Autodesk Fusion 360 part; units mm, degrees
(part 3 of 8)
  line L38 (161.2459, -8.965) -> (161.2459, 4.1583)
  spline S145 degree 3 poles (161.2459, 4.1583) (161.2459, 5.296) (159.7907, 5.2166) (159.7907, 5.6135) knots 0 0 0 0 1 1 1 1
  spline S146 degree 3 poles (159.7907, 5.6135) (159.7907, 5.9575) (160.0818, 6.5131) (160.2934, 6.5131) knots 0 0 0 0 1 1 1 1
  spline S147 degree 3 poles (160.2934, 6.5131) (161.3253, 6.4602) (162.6218, 6.4337) (163.9182, 6.4337) knots 0 0 0 0 1 1 1 1
  spline S148 degree 3 poles (163.9182, 6.4337) (165.2147, 6.4337) (166.4873, 6.4602) (167.5457, 6.5131) knots 0 0 0 0 1 1 1 1
  spline S149 degree 3 poles (167.5457, 6.5131) (167.7547, 6.5131) (168.0193, 5.9575) (168.0193, 5.64) knots 0 0 0 0 1 1 1 1
  spline S150 degree 3 poles (168.0193, 5.64) (168.0193, 5.2166) (166.5905, 5.296) (166.5905, 4.1583) knots 0 0 0 0 1 1 1 1
  line L39 (166.5905, 4.1583) -> (166.5905, -8.965)
  spline S151 degree 3 poles (166.5905, -8.965) (166.5905, -10.0763) (168.0193, -10.0234) (168.0193, -10.4203) knots 0 0 0 0 1 1 1 1
  spline S152 degree 3 poles (168.0193, -10.4203) (168.0193, -10.7378) (167.7547, -11.3225) (167.5457, -11.2934) knots 0 0 0 0 1 1 1 1
  spline S153 degree 3 poles (167.5457, -11.2934) (166.4873, -11.2405) (165.2147, -11.214) (163.9182, -11.214) knots 0 0 0 0 1 1 1 1
  spline S154 degree 3 poles (163.9182, -11.214) (162.6218, -11.214) (161.3253, -11.2405) (160.2934, -11.2934) knots 0 0 0 0 1 1 1 1
  spline S155 degree 3 poles (160.2934, -11.2934) (160.0818, -11.3225) (159.7907, -10.7378) (159.7907, -10.4203) knots 0 0 0 0 1 1 1 1
  spline S156 degree 3 poles (-72.8517, 6.434) (-72.0838, 6.434) (-71.3407, 6.4603) (-70.4164, 6.5133) knots 0 0 0 0 1 1 1 1
  spline S157 degree 3 poles (-70.4164, 6.5133) (-71.3407, 6.4603) (-72.0838, 6.434) (-72.8517, 6.434) knots -1 -1 -1 -1 0 0 0 0
  spline S158 degree 3 poles (9.5118, 5.6398) (9.5118, 5.2165) (8.0583, 5.2959) (8.0583, 4.1848) knots 0 0 0 0 1 1 1 1
  spline S159 degree 3 poles (8.0583, 4.1848) (8.0583, 5.2959) (9.5118, 5.2165) (9.5118, 5.6398) knots -1 -1 -1 -1 0 0 0 0
  spline S160 degree 3 poles (159.7907, -10.4203) (159.7907, -10.0234) (161.2459, -10.0763) (161.2459, -8.965) knots 0 0 0 0 1 1 1 1
  spline S161 degree 3 poles (161.2459, -8.965) (161.2459, -10.0763) (159.7907, -10.0234) (159.7907, -10.4203) knots -1 -1 -1 -1 0 0 0 0
  spline S162 degree 3 poles (88.5675, 6.5131) (88.9644, 6.4602) (90.5519, 6.4337) (92.1394, 6.4337) knots 0 0 0 0 1 1 1 1
  spline S163 degree 3 poles (92.1394, 6.4337) (90.5519, 6.4337) (88.9644, 6.4602) (88.5675, 6.5131) knots -1 -1 -1 -1 0 0 0 0
  line L40 (2.7113, 4.1848) -> (2.7113, -0.5248)
  line L41 (2.7113, -0.5248) -> (2.7113, 4.1848)
  spline S164 degree 3 poles (161.2459, -8.965) (161.2459, -10.0763) (159.7907, -10.0234) (159.7907, -10.4203) knots -1 -1 -1 -1 0 0 0 0
  spline S165 degree 3 poles (159.7907, -10.4203) (159.7907, -10.7378) (160.0818, -11.3225) (160.2934, -11.2934) knots -1 -1 -1 -1 0 0 0 0
  spline S166 degree 3 poles (160.2934, -11.2934) (161.3253, -11.2405) (162.6218, -11.214) (163.9182, -11.214) knots -1 -1 -1 -1 0 0 0 0
  spline S167 degree 3 poles (163.9182, -11.214) (165.2147, -11.214) (166.4873, -11.2405) (167.5457, -11.2934) knots -1 -1 -1 -1 0 0 0 0
  spline S168 degree 3 poles (167.5457, -11.2934) (167.7547, -11.3225) (168.0193, -10.7378) (168.0193, -10.4203) knots -1 -1 -1 -1 0 0 0 0
  spline S169 degree 3 poles (168.0193, -10.4203) (168.0193, -10.0234) (166.5905, -10.0763) (166.5905, -8.965) knots -1 -1 -1 -1 0 0 0 0
  line L42 (166.5905, -8.965) -> (166.5905, 4.1583)
  spline S170 degree 3 poles (166.5905, 4.1583) (166.5905, 5.296) (168.0193, 5.2166) (168.0193, 5.64) knots -1 -1 -1 -1 0 0 0 0
  spline S171 degree 3 poles (168.0193, 5.64) (168.0193, 5.9575) (167.7547, 6.5131) (167.5457, 6.5131) knots -1 -1 -1 -1 0 0 0 0
  spline S172 degree 3 poles (167.5457, 6.5131) (166.4873, 6.4602) (165.2147, 6.4337) (163.9182, 6.4337) knots -1 -1 -1 -1 0 0 0 0
  spline S173 degree 3 poles (163.9182, 6.4337) (162.6218, 6.4337) (161.3253, 6.4602) (160.2934, 6.5131) knots -1 -1 -1 -1 0 0 0 0
  spline S174 degree 3 poles (160.2934, 6.5131) (160.0818, 6.5131) (159.7907, 5.9575) (159.7907, 5.6135) knots -1 -1 -1 -1 0 0 0 0
  spline S175 degree 3 poles (159.7907, 5.6135) (159.7907, 5.2166) (161.2459, 5.296) (161.2459, 4.1583) knots -1 -1 -1 -1 0 0 0 0
  line L43 (161.2459, 4.1583) -> (161.2459, -8.965)
  spline S176 degree 3 poles (112.1948, 6.5131) (112.4065, 6.5395) (112.6975, 5.931) (112.6975, 5.6135) knots 0 0 0 0 1 1 1 1
  spline S177 degree 3 poles (112.6975, 5.6135) (112.6975, 5.931) (112.4065, 6.5395) (112.1948, 6.5131) knots -1 -1 -1 -1 0 0 0 0
  spline S178 degree 3 poles (109.7077, -8.9386) (109.5755, -10.0498) (111.2952, -9.9969) (111.2952, -10.4203) knots 0 0 0 0 1 1 1 1
  spline S179 degree 3 poles (111.2952, -10.4203) (111.2952, -9.9969) (109.5755, -10.0498) (109.7077, -8.9386) knots -1 -1 -1 -1 0 0 0 0
  spline S180 degree 3 poles (8.0583, -8.9652) (8.0583, -10.0763) (9.5118, -9.9969) (9.5118, -10.4202) knots 0 0 0 0 1 1 1 1
  spline S181 degree 3 poles (9.5118, -10.4202) (9.5118, -9.9969) (8.0583, -10.0763) (8.0583, -8.9652) knots -1 -1 -1 -1 0 0 0 0
  spline S182 degree 3 poles (166.5905, -8.965) (166.5905, -10.0763) (168.0193, -10.0234) (168.0193, -10.4203) knots 0 0 0 0 1 1 1 1
  spline S183 degree 3 poles (168.0193, -10.4203) (168.0193, -10.0234) (166.5905, -10.0763) (166.5905, -8.965) knots -1 -1 -1 -1 0 0 0 0
  line L44 (111.3746, 4.1583) -> (109.7077, -8.9386)
  spline S184 degree 3 poles (109.7077, -8.9386) (109.5755, -10.0498) (111.2952, -9.9969) (111.2952, -10.4203) knots 0 0 0 0 1 1 1 1
  spline S185 degree 3 poles (111.2952, -10.4203) (111.2952, -10.7378) (111.0042, -11.3225) (110.7925, -11.2934) knots 0 0 0 0 1 1 1 1
  spline S186 degree 3 poles (110.7925, -11.2934) (108.914, -11.1346) (106.9032, -11.2934) (106.0036, -11.2934) knots 0 0 0 0 1 1 1 1
  spline S187 degree 3 poles (106.0036, -11.2934) (105.104, -11.2934) (104.8394, -11.1346) (104.6542, -10.6584) knots 0 0 0 0 1 1 1 1
  line L45 (104.6542, -10.6584) -> (100.1563, 1.6977)
  line L46 (100.1563, 1.6977) -> (95.6584, -10.6584)
  spline S188 degree 3 poles (95.6584, -10.6584) (95.4732, -11.1346) (95.235, -11.2934) (94.309, -11.2934) knots 0 0 0 0 1 1 1 1
  spline S189 degree 3 poles (94.309, -11.2934) (93.4094, -11.2934) (91.6367, -11.1346) (89.7317, -11.2934) knots 0 0 0 0 1 1 1 1
  spline S190 degree 3 poles (89.7317, -11.2934) (89.52, -11.3225) (89.2555, -10.7378) (89.2555, -10.4203) knots 0 0 0 0 1 1 1 1
  spline S191 degree 3 poles (89.2555, -10.4203) (89.2555, -9.9969) (90.9223, -10.0234) (90.8165, -8.9121) knots 0 0 0 0 1 1 1 1
  line L47 (90.8165, -8.9121) -> (89.3877, 4.1583)
  spline S192 degree 3 poles (89.3877, 4.1583) (89.2819, 5.296) (88.0913, 5.2166) (88.0913, 5.6135) knots 0 0 0 0 1 1 1 1
  spline S193 degree 3 poles (88.0913, 5.6135) (88.0913, 5.931) (88.3559, 6.5395) (88.5675, 6.5131) knots 0 0 0 0 1 1 1 1
  spline S194 degree 3 poles (88.5675, 6.5131) (88.9644, 6.4602) (90.5519, 6.4337) (92.1394, 6.4337) knots 0 0 0 0 1 1 1 1
  spline S195 degree 3 poles (92.1394, 6.4337) (93.7005, 6.4337) (95.288, 6.4602) (95.6848, 6.5131) knots 0 0 0 0 1 1 1 1
  spline S196 degree 3 poles (95.6848, 6.5131) (95.8965, 6.5395) (96.1875, 5.931) (96.1875, 5.6135) knots 0 0 0 0 1 1 1 1
  spline S197 degree 3 poles (96.1875, 5.6135) (96.1875, 5.2166) (94.6265, 5.296) (94.7323, 4.1583) knots 0 0 0 0 1 1 1 1
  line L48 (94.7323, 4.1583) -> (95.7113, -4.7053)
  line L49 (95.7113, -4.7053) -> (99.7859, 6.5131)
  spline S198 degree 3 poles (99.7859, 6.5131) (100.6855, 6.4602) (101.3469, 6.4337) (102.0084, 6.4337) knots 0 0 0 0 1 1 1 1
  spline S199 degree 3 poles (102.0084, 6.4337) (102.6698, 6.4337) (103.3313, 6.4602) (104.2573, 6.5131) knots 0 0 0 0 1 1 1 1
  line L50 (104.2573, 6.5131) -> (108.2261, -4.7317)
  line L51 (108.2261, -4.7317) -> (109.3902, 4.1583)
  spline S200 degree 3 poles (109.3902, 4.1583) (109.549, 5.296) (107.9615, 5.2166) (107.9615, 5.6135) knots 0 0 0 0 1 1 1 1
  spline S201 degree 3 poles (107.9615, 5.6135) (107.9615, 5.931) (108.2261, 6.5395) (108.4377, 6.5131) knots 0 0 0 0 1 1 1 1
  spline S202 degree 3 poles (108.4377, 6.5131) (108.8346, 6.4602) (109.5755, 6.4337) (110.3163, 6.4337) knots 0 0 0 0 1 1 1 1
  spline S203 degree 3 poles (110.3163, 6.4337) (111.0571, 6.4337) (111.798, 6.4602) (112.1948, 6.5131) knots 0 0 0 0 1 1 1 1
  spline S204 degree 3 poles (112.1948, 6.5131) (112.4065, 6.5395) (112.6975, 5.931) (112.6975, 5.6135) knots 0 0 0 0 1 1 1 1
  spline S205 degree 3 poles (112.6975, 5.6135) (112.6975, 5.2166) (111.5334, 5.296) (111.3746, 4.1583) knots 0 0 0 0 1 1 1 1
  line L52 (109.7077, -8.9386) -> (111.3746, 4.1583)
  line L53 (111.3746, 4.1583) -> (109.7077, -8.9386)
  line L54 (2.7113, -0.5248) -> (0.9622, -0.5248)
  line L55 (0.9622, -0.5248) -> (2.7113, -0.5248)
  spline S206 degree 3 poles (107.9615, 5.6135) (107.9615, 5.931) (108.2261, 6.5395) (108.4377, 6.5131) knots 0 0 0 0 1 1 1 1
  spline S207 degree 3 poles (108.4377, 6.5131) (108.2261, 6.5395) (107.9615, 5.931) (107.9615, 5.6135) knots -1 -1 -1 -1 0 0 0 0
  spline S208 degree 3 poles (9.5118, -10.4202) (9.5118, -10.738) (9.2223, -11.3225) (9.0107, -11.2935) knots 0 0 0 0 1 1 1 1
  spline S209 degree 3 poles (9.0107, -11.2935) (9.2223, -11.3225) (9.5118, -10.738) (9.5118, -10.4202) knots -1 -1 -1 -1 0 0 0 0
  spline S210 degree 3 poles (214.7182, 6.5131) (215.7501, 6.4602) (217.0466, 6.4337) (218.3166, 6.4337) knots 0 0 0 0 1 1 1 1
  spline S211 degree 3 poles (218.3166, 6.4337) (217.0466, 6.4337) (215.7501, 6.4602) (214.7182, 6.5131) knots -1 -1 -1 -1 0 0 0 0
  spline S212 degree 3 poles (111.2952, -10.4203) (111.2952, -10.7378) (111.0042, -11.3225) (110.7925, -11.2934) knots 0 0 0 0 1 1 1 1
  spline S213 degree 3 poles (110.7925, -11.2934) (111.0042, -11.3225) (111.2952, -10.7378) (111.2952, -10.4203) knots -1 -1 -1 -1 0 0 0 0
  spline S214 degree 3 poles (168.0193, -10.4203) (168.0193, -10.7378) (167.7547, -11.3225) (167.5457, -11.2934) knots 0 0 0 0 1 1 1 1
  spline S215 degree 3 poles (167.5457, -11.2934) (167.7547, -11.3225) (168.0193, -10.7378) (168.0193, -10.4203) knots -1 -1 -1 -1 0 0 0 0
  spline S216 degree 3 poles (207.4951, -6.769) (207.4951, -6.5573) (208.0507, -6.2663) (208.3682, -6.2663) knots 0 0 0 0 1 1 1 1
  spline S217 degree 3 poles (208.3682, -6.2663) (208.0507, -6.2663) (207.4951, -6.5573) (207.4951, -6.769) knots -1 -1 -1 -1 0 0 0 0
  spline S218 degree 3 poles (108.4377, 6.5131) (108.8346, 6.4602) (109.5755, 6.4337) (110.3163, 6.4337) knots 0 0 0 0 1 1 1 1
  spline S219 degree 3 poles (110.3163, 6.4337) (109.5755, 6.4337) (108.8346, 6.4602) (108.4377, 6.5131) knots -1 -1 -1 -1 0 0 0 0
  line L56 (215.6707, -3.1442) -> (215.6707, -8.7798)
  line L57 (215.6707, -8.7798) -> (215.6707, -3.1442)
  line L58 (-61.1571, -8.9652) -> (-61.1571, -0.6308)
  spline S220 degree 3 poles (-61.1571, -0.6308) (-61.1571, 4.158) (-58.5644, 6.7775) (-53.9628, 6.7775) knots 0 0 0 0 0.999995 0.999995 0.999995 0.999995
  line L59 (-53.9628, 6.7775) -> (-53.9628, 6.7775)
  spline S221 degree 3 poles (-53.9628, 6.7775) (-49.3578, 6.7775) (-46.7651, 4.158) (-46.7651, -0.6308) knots 0.000005 0.000005 0.000005 0.000005 1 1 1 1
  line L60 (-46.7651, -0.6308) -> (-46.7651, -8.9652)
  spline S222 degree 3 poles (-46.7651, -8.9652) (-46.7651, -10.0765) (-45.3365, -9.9971) (-45.3365, -10.4202) knots 0 0 0 0 1 1 1 1
  spline S223 degree 3 poles (-45.3365, -10.4202) (-45.3365, -10.7379) (-45.601, -11.2935) (-45.8379, -11.2935) knots 0 0 0 0 1 1 1 1
  ellipse E6 centre (-50.1303, -11.6956) end of major axis (-56.9584, -11.7428) minor radius 0.4792 (-45.8379, -11.2935) -> (-49.4642, -11.2142) ccw
  ellipse E7 centre (-49.574, -11.5198) end of major axis (-54.89, -11.5263) minor radius 0.3056 (-49.4642, -11.2142) -> (-53.0631, -11.2935) ccw
  spline S224 degree 3 poles (-53.0631, -11.2935) (-53.2726, -11.2935) (-53.5645, -10.7379) (-53.5645, -10.4202) knots 0 0 0 0 1 1 1 1
  spline S225 degree 3 poles (-53.5645, -10.4202) (-53.5645, -9.9971) (-52.1084, -10.0765) (-52.1084, -8.9652) knots 0 0 0 0 1 1 1 1
  line L61 (-52.1084, -8.9652) -> (-52.1084, -0.3134)
  spline S226 degree 3 poles (-52.1084, -0.3134) (-52.1084, 2.7559) (-53.434, 4.3435) (-55.6798, 4.3435) knots 0 0 0 0 1 1 1 1
  spline S227 degree 3 poles (-55.6798, 4.3435) (-57.9291, 4.3435) (-59.2547, 2.7559) (-59.2547, -0.3134) knots 0 0 0 0 1 1 1 1
  line L62 (-59.2547, -0.3134) -> (-59.2547, -8.9652)
  spline S228 degree 3 poles (-59.2547, -8.9652) (-59.2547, -10.0765) (-57.7986, -9.9971) (-57.7986, -10.4202) knots 0 0 0 0 1 1 1 1
  spline S229 degree 3 poles (-57.7986, -10.4202) (-57.7986, -10.7379) (-58.0905, -11.3227) (-58.3, -11.2935) knots 0 0 0 0 1 1 1 1
  ellipse E8 centre (-60.2658, -11.5026) end of major axis (-63.0589, -11.5087) minor radius 0.2884 (-58.3, -11.2935) -> (-60.2059, -11.2142) ccw
  ellipse E9 centre (-60.1459, -11.5026) end of major axis (-62.939, -11.4965) minor radius 0.2884 (-60.2059, -11.2142) -> (-62.1118, -11.2935) ccw
  spline S230 degree 3 poles (-62.1118, -11.2935) (-62.3212, -11.3227) (-62.5342, -10.7379) (-62.5342, -10.4202) knots 0 0 0 0 1 1 1 1
  spline S231 degree 3 poles (-62.5342, -10.4202) (-62.5342, -9.9971) (-61.1571, -10.0765) (-61.1571, -8.9652) knots 0 0 0 0 1 1 1 1
  spline S232 degree 3 poles (-11.2033, 5.6928) (-11.0976, 5.2958) (-10.2518, 1.4065) (-10.2518, 1.195) knots 0 0 0 0 1 1 1 1
  spline S233 degree 3 poles (-10.2518, 1.195) (-10.2518, 1.4065) (-11.0976, 5.2958) (-11.2033, 5.6928) knots -1 -1 -1 -1 0 0 0 0
  spline S234 degree 3 poles (311.924, 6.4866) (312.3209, 6.4337) (313.1149, 6.4072) (313.9086, 6.4072) knots 0 0 0 0 1 1 1 1
  spline S235 degree 3 poles (313.9086, 6.4072) (313.1149, 6.4072) (312.3209, 6.4337) (311.924, 6.4866) knots -1 -1 -1 -1 0 0 0 0
  line L63 (-61.1571, -0.6308) -> (-61.1571, -8.9652)
  line L64 (-61.1571, -8.9652) -> (-61.1571, -0.6308)
  ellipse E10 centre (19.5885, -1.7408) end of major axis (19.5885, -11.5568) minor radius 8.5372 (12.3354, 3.4367) -> (19.0342, -11.5361) ccw
  ellipse E11 centre (19.5885, -1.7408) end of major axis (19.5885, -11.5568) minor radius 8.5372 (12.3354, 3.4367) -> (19.0342, -11.5361) ccw
  spline S236 degree 3 poles (-35.3861, -11.2138) (-38.111, -11.2138) (-40.8658, -11.2404) (-43.5907, -11.2933) knots 0 0 0 0 1 1 1 1
  spline S237 degree 3 poles (-43.5907, -11.2933) (-40.8658, -11.2404) (-38.111, -11.2138) (-35.3861, -11.2138) knots -1 -1 -1 -1 0 0 0 0
  spline S238 degree 3 poles (16.2828, -2.3771) (16.2828, 2.518) (17.3668, 4.9254) (19.7498, 4.9254) knots -1 -1 -1 -1 0 0 0 0
  spline S239 degree 3 poles (16.2828, -2.3771) (16.2828, 2.518) (17.3668, 4.9254) (19.7498, 4.9254) knots -1 -1 -1 -1 0 0 0 0
  spline S240 degree 3 poles (-37.7953, 4.1582) (-37.7953, 5.296) (-39.2508, 5.2166) (-39.2508, 5.6137) knots 0 0 0 0 1 1 1 1
  spline S241 degree 3 poles (-39.2508, 5.6137) (-39.2508, 5.2166) (-37.7953, 5.296) (-37.7953, 4.1582) knots -1 -1 -1 -1 0 0 0 0
  spline S242 degree 3 poles (18.0029, 6.6455) (17.2638, 6.85) (16.5713, 7.0359) (15.9755, 7.1529) knots 0 0 0 0 0.594925 0.594925 0.594925 0.594925
  spline S243 degree 3 poles (15.9755, 7.1529) (16.5713, 7.0359) (17.2638, 6.85) (18.0029, 6.6455) knots -0.594925 -0.594925 -0.594925 -0.594925 0 0 0 0
  spline S244 degree 3 poles (-43.5907, -11.2933) (-44.1191, -11.3225) (-44.4381, -11.161) (-44.4381, -10.6848) knots 0 0 0 0 1 1 1 1
  spline S245 degree 3 poles (-44.4381, -10.6848) (-44.4381, -11.161) (-44.1191, -11.3225) (-43.5907, -11.2933) knots -1 -1 -1 -1 0 0 0 0
  spline S246 degree 3 poles (24.3546, 13.0748) (26.2837, 13.0748) (27.8455, 11.3814) (27.8455, 9.3176) knots 0 0 0 0 1 1 1 1
  spline S247 degree 3 poles (27.8455, 9.3176) (27.8455, 11.3814) (26.2837, 13.0748) (24.3546, 13.0748) knots -1 -1 -1 -1 0 0 0 0
  spline S248 degree 3 poles (-39.2508, 5.6137) (-39.2508, 5.931) (-38.9584, 6.5132) (-38.7457, 6.5132) knots 0 0 0 0 1 1 1 1
  spline S249 degree 3 poles (-38.7457, 6.5132) (-38.9584, 6.5132) (-39.2508, 5.931) (-39.2508, 5.6137) knots -1 -1 -1 -1 0 0 0 0
  spline S250 degree 3 poles (15.9755, 7.1529) (15.5699, 7.2326) (15.2092, 7.2804) (14.9092, 7.2804) knots 0.594925 0.594925 0.594925 0.594925 1 1 1 1
  spline S251 degree 3 poles (14.9092, 7.2804) (15.2092, 7.2804) (15.5699, 7.2326) (15.9755, 7.1529) knots -1 -1 -1 -1 -0.594925 -0.594925 -0.594925 -0.594925
  spline S252 degree 3 poles (-44.4381, -10.6848) (-44.4381, -10.1292) (-44.0427, -6.4516) (-44.0427, -6.2399) knots 0 0 0 0 1 1 1 1
  spline S253 degree 3 poles (-44.0427, -6.2399) (-44.0427, -6.4516) (-44.4381, -10.1292) (-44.4381, -10.6848) knots -1 -1 -1 -1 0 0 0 0
  spline S254 degree 3 poles (-38.7457, 6.5132) (-37.7156, 6.46) (-36.4196, 6.4338) (-35.1236, 6.4338) knots 0 0 0 0 1 1 1 1
  spline S255 degree 3 poles (-35.1236, 6.4338) (-36.4196, 6.4338) (-37.7156, 6.46) (-38.7457, 6.5132) knots -1 -1 -1 -1 0 0 0 0
  spline S256 degree 3 poles (21.3624, 10.7728) (21.3624, 11.8842) (22.739, 13.0748) (24.3546, 13.0748) knots 0 0 0 0 1 1 1 1
  spline S257 degree 3 poles (24.3546, 13.0748) (22.739, 13.0748) (21.3624, 11.8842) (21.3624, 10.7728) knots -1 -1 -1 -1 0 0 0 0
  spline S258 degree 3 poles (-27.1849, -11.2933) (-29.9364, -11.2404) (-32.6613, -11.2138) (-35.3861, -11.2138) knots 0 0 0 0 1 1 1 1
  spline S259 degree 3 poles (-35.3861, -11.2138) (-32.6613, -11.2138) (-29.9364, -11.2404) (-27.1849, -11.2933) knots -1 -1 -1 -1 0 0 0 0
  spline S260 degree 3 poles (14.9092, 7.2804) (13.9565, 7.2804) (13.637, 6.8569) (13.637, 6.2749) knots 0 0 0 0 1 1 1 1
  spline S261 degree 3 poles (13.637, 6.2749) (13.637, 6.8569) (13.9565, 7.2804) (14.9092, 7.2804) knots -1 -1 -1 -1 0 0 0 0
  spline S262 degree 3 poles (22.8466, 8.9736) (22.2105, 8.9736) (21.3624, 9.9262) (21.3624, 10.7728) knots 0 0 0 0 1 1 1 1
  spline S263 degree 3 poles (21.3624, 10.7728) (21.3624, 9.9262) (22.2105, 8.9736) (22.8466, 8.9736) knots -1 -1 -1 -1 0 0 0 0
  spline S264 degree 3 poles (-35.1236, 6.4338) (-33.8243, 6.4338) (-32.5549, 6.46) (-31.4982, 6.5132) knots 0 0 0 0 1 1 1 1
  spline S265 degree 3 poles (-31.4982, 6.5132) (-32.5549, 6.46) (-33.8243, 6.4338) (-35.1236, 6.4338) knots -1 -1 -1 -1 0 0 0 0
  spline S266 degree 3 poles (13.637, 6.2749) (13.637, 6.2221) (13.5056, 6.1955) (13.3205, 6.1955) knots 0 0 0 0 1 1 1 1
  spline S267 degree 3 poles (13.3205, 6.1955) (13.5056, 6.1955) (13.637, 6.2221) (13.637, 6.2749) knots -1 -1 -1 -1 0 0 0 0
  spline S268 degree 3 poles (24.0351, 9.5293) (23.3482, 9.5293) (23.0556, 8.9736) (22.8466, 8.9736) knots 0 0 0 0 1 1 1 1
  spline S269 degree 3 poles (22.8466, 8.9736) (23.0556, 8.9736) (23.3482, 9.5293) (24.0351, 9.5293) knots -1 -1 -1 -1 0 0 0 0
  spline S270 degree 3 poles (-26.2578, -10.4731) (-26.3641, -11.161) (-26.63, -11.3225) (-27.1849, -11.2933) knots 0 0 0 0 1 1 1 1
  spline S271 degree 3 poles (-27.1849, -11.2933) (-26.63, -11.3225) (-26.3641, -11.161) (-26.2578, -10.4731) knots -1 -1 -1 -1 0 0 0 0
  spline S272 degree 3 poles (109.3902, 4.1583) (109.549, 5.296) (107.9615, 5.2166) (107.9615, 5.6135) knots 0 0 0 0 1 1 1 1
  spline S273 degree 3 poles (107.9615, 5.6135) (107.9615, 5.2166) (109.549, 5.296) (109.3902, 4.1583) knots -1 -1 -1 -1 0 0 0 0
  spline S274 degree 3 poles (215.6707, -8.7798) (215.6707, -9.4148) (215.3268, -9.3619) (213.7393, -9.3619) knots -1 -1 -1 -1 0 0 0 0
  spline S275 degree 3 poles (213.7393, -9.3619) (208.9503, -9.3619) (208.8709, -6.2663) (208.3682, -6.2663) knots -1 -1 -1 -1 0 0 0 0
  spline S276 degree 3 poles (208.3682, -6.2663) (208.0507, -6.2663) (207.4951, -6.5573) (207.4951, -6.769) knots -1 -1 -1 -1 0 0 0 0
  spline S277 degree 3 poles (207.4951, -6.769) (207.4951, -6.9807) (207.0718, -10.1028) (207.0718, -10.6848) knots -1 -1 -1 -1 0 0 0 0
  spline S278 degree 3 poles (207.0718, -10.6848) (207.0718, -11.1611) (207.3893, -11.3225) (207.9184, -11.2934) knots -1 -1 -1 -1 0 0 0 0
  spline S279 degree 3 poles (207.9184, -11.2934) (209.8764, -11.2405) (212.628, -11.214) (215.3532, -11.214) knots -1 -1 -1 -1 0 0 0 0
  spline S280 degree 3 poles (215.3532, -11.214) (217.7874, -11.214) (220.1951, -11.2405) (221.9414, -11.2934) knots -1 -1 -1 -1 0 0 0 0
  spline S281 degree 3 poles (221.9414, -11.2934) (222.1795, -11.2934) (222.4441, -10.7113) (222.4441, -10.3938) knots -1 -1 -1 -1 0 0 0 0
  spline S282 degree 3 poles (222.4441, -10.3938) (222.4441, -9.9969) (221.0153, -10.0763) (221.0153, -8.9386) knots -1 -1 -1 -1 0 0 0 0
  line L65 (221.0153, -8.9386) -> (221.0153, 4.1583)
  spline S283 degree 3 poles (221.0153, 4.1583) (221.0153, 5.296) (222.4441, 5.2166) (222.4441, 5.64) knots -1 -1 -1 -1 0 0 0 0
  spline S284 degree 3 poles (222.4441, 5.64) (222.4441, 5.9575) (222.1795, 6.5131) (221.9414, 6.5131) knots -1 -1 -1 -1 0 0 0 0
  spline S285 degree 3 poles (221.9414, 6.5131) (220.883, 6.4602) (219.613, 6.4337) (218.3166, 6.4337) knots -1 -1 -1 -1 0 0 0 0
  spline S286 degree 3 poles (218.3166, 6.4337) (217.0466, 6.4337) (215.7501, 6.4602) (214.7182, 6.5131) knots -1 -1 -1 -1 0 0 0 0
  spline S287 degree 3 poles (214.7182, 6.5131) (214.5066, 6.5131) (214.2155, 5.9575) (214.2155, 5.6135) knots -1 -1 -1 -1 0 0 0 0
  spline S288 degree 3 poles (214.2155, 5.6135) (214.2155, 5.2166) (215.6707, 5.296) (215.6707, 4.1583) knots -1 -1 -1 -1 0 0 0 0
  line L66 (215.6707, 4.1583) -> (215.6707, -1.2921)
  line L67 (215.6707, -1.2921) -> (213.8186, -1.2392)
  spline S289 degree 3 poles (213.8186, -1.2392) (211.6491, -1.1863) (211.8078, 1.5389) (211.0141, 1.5389) knots -1 -1 -1 -1 0 0 0 0
  spline S290 degree 3 poles (211.0141, 1.5389) (210.6966, 1.5389) (210.1145, 1.2479) (210.1145, 1.0362) knots -1 -1 -1 -1 0 0 0 0
  spline S291 degree 3 poles (210.1145, 1.0362) (210.2468, -1.1334) (210.2468, -3.303) (210.1145, -5.4725) knots -1 -1 -1 -1 0 0 0 0
  spline S292 degree 3 poles (210.1145, -5.4725) (210.1145, -5.6842) (210.6966, -5.9753) (211.0141, -5.9753) knots -1 -1 -1 -1 0 0 0 0
  spline S293 degree 3 poles (211.0141, -5.9753) (211.8078, -5.9753) (211.6491, -3.25) (213.8186, -3.1971) knots -1 -1 -1 -1 0 0 0 0
  line L68 (213.8186, -3.1971) -> (215.6707, -3.1442)
  line L69 (215.6707, -3.1442) -> (215.6707, -8.7798)
  line L70 (100.1563, 1.6977) -> (104.6542, -10.6584)
  line L71 (104.6542, -10.6584) -> (100.1563, 1.6977)
  spline S294 degree 3 poles (313.9086, 6.4072) (314.7024, 6.4072) (315.4961, 6.4337) (315.893, 6.4866) knots 0 0 0 0 1 1 1 1
  spline S295 degree 3 poles (315.893, 6.4866) (315.4961, 6.4337) (314.7024, 6.4072) (313.9086, 6.4072) knots -1 -1 -1 -1 0 0 0 0
  spline S296 degree 3 poles (-17.4217, 6.7775) (-14.9356, 6.7775) (-14.1155, 6.2749) (-13.1896, 6.2749) knots 0 0 0 0 1 1 1 1
  spline S297 degree 3 poles (-13.1896, 6.2749) (-14.1155, 6.2749) (-14.9356, 6.7775) (-17.4217, 6.7775) knots -1 -1 -1 -1 0 0 0 0
  line L72 (-61.1571, -0.6308) -> (-61.1571, -8.9652)
  spline S298 degree 3 poles (-61.1571, -8.9652) (-61.1571, -10.0765) (-62.5342, -9.9971) (-62.5342, -10.4202) knots -1 -1 -1 -1 0 0 0 0
  spline S299 degree 3 poles (-62.5342, -10.4202) (-62.5342, -10.7379) (-62.3212, -11.3227) (-62.1118, -11.2935) knots -1 -1 -1 -1 0 0 0 0
  ellipse E12 centre (-60.1459, -11.5026) end of major axis (-62.939, -11.4965) minor radius 0.2884 (-60.2059, -11.2142) -> (-62.1118, -11.2935) ccw
  ellipse E13 centre (-60.2658, -11.5026) end of major axis (-63.0589, -11.5087) minor radius 0.2884 (-58.3, -11.2935) -> (-60.2059, -11.2142) ccw
  spline S300 degree 3 poles (-58.3, -11.2935) (-58.0905, -11.3227) (-57.7986, -10.7379) (-57.7986, -10.4202) knots -1 -1 -1 -1 0 0 0 0
  spline S301 degree 3 poles (-57.7986, -10.4202) (-57.7986, -9.9971) (-59.2547, -10.0765) (-59.2547, -8.9652) knots -1 -1 -1 -1 0 0 0 0
  line L73 (-59.2547, -8.9652) -> (-59.2547, -0.3134)
  spline S302 degree 3 poles (-59.2547, -0.3134) (-59.2547, 2.7559) (-57.9291, 4.3435) (-55.6798, 4.3435) knots -1 -1 -1 -1 0 0 0 0
  spline S303 degree 3 poles (-55.6798, 4.3435) (-53.434, 4.3435) (-52.1084, 2.7559) (-52.1084, -0.3134) knots -1 -1 -1 -1 0 0 0 0
  line L74 (-52.1084, -0.3134) -> (-52.1084, -8.9652)
  spline S304 degree 3 poles (-52.1084, -8.9652) (-52.1084, -10.0765) (-53.5645, -9.9971) (-53.5645, -10.4202) knots -1 -1 -1 -1 0 0 0 0
  spline S305 degree 3 poles (-53.5645, -10.4202) (-53.5645, -10.7379) (-53.2726, -11.2935) (-53.0631, -11.2935) knots -1 -1 -1 -1 0 0 0 0
  ellipse E14 centre (-49.574, -11.5198) end of major axis (-54.89, -11.5263) minor radius 0.3056 (-49.4642, -11.2142) -> (-53.0631, -11.2935) ccw
  ellipse E15 centre (-50.1303, -11.6956) end of major axis (-56.9584, -11.7428) minor radius 0.4792 (-45.8379, -11.2935) -> (-49.4642, -11.2142) ccw
  spline S306 degree 3 poles (-45.8379, -11.2935) (-45.601, -11.2935) (-45.3365, -10.7379) (-45.3365, -10.4202) knots -1 -1 -1 -1 0 0 0 0
  spline S307 degree 3 poles (-45.3365, -10.4202) (-45.3365, -9.9971) (-46.7651, -10.0765) (-46.7651, -8.9652) knots -1 -1 -1 -1 0 0 0 0
  line L75 (-46.7651, -8.9652) -> (-46.7651, -0.6308)
  spline S308 degree 3 poles (-46.7651, -0.6308) (-46.7651, 4.158) (-49.3578, 6.7775) (-53.9628, 6.7775) knots -1 -1 -1 -1 -0.000005 -0.000005 -0.000005 -0.000005
  line L76 (-53.9628, 6.7775) -> (-53.9628, 6.7775)
  spline S309 degree 3 poles (-53.9628, 6.7775) (-58.5644, 6.7775) (-61.1571, 4.158) (-61.1571, -0.6308) knots -0.999995 -0.999995 -0.999995 -0.999995 0 0 0 0
  line L77 (299.0115, 4.1318) -> (304.277, -10.6848)
  line L78 (304.277, -10.6848) -> (299.0115, 4.1318)
  spline S310 degree 3 poles (-115.636, 5.6133) (-115.636, 5.2164) (-116.5623, 5.0843) (-117.1979, 4.132) knots 0 0 0 0 1 1 1 1
  spline S311 degree 3 poles (-117.1979, 4.132) (-116.5623, 5.0843) (-115.636, 5.2164) (-115.636, 5.6133) knots -1 -1 -1 -1 0 0 0 0
  spline S312 degree 3 poles (110.7925, -11.2934) (108.914, -11.1346) (106.9032, -11.2934) (106.0036, -11.2934) knots 0 0 0 0 1 1 1 1
  spline S313 degree 3 poles (106.0036, -11.2934) (106.9032, -11.2934) (108.914, -11.1346) (110.7925, -11.2934) knots -1 -1 -1 -1 0 0 0 0
  line L79 (-64.9913, -8.9383) -> (-70.4164, 6.5133)
  spline S314 degree 3 poles (-70.4164, 6.5133) (-71.3407, 6.4603) (-72.0838, 6.434) (-72.8517, 6.434) knots -1 -1 -1 -1 0 0 0 0
  spline S315 degree 3 poles (-72.8517, 6.434) (-73.5911, 6.434) (-74.3591, 6.4603) (-75.2585, 6.5133) knots -1 -1 -1 -1 0 0 0 0
  line L80 (-75.2585, 6.5133) -> (-80.6801, -8.9383)
  spline S316 degree 3 poles (-80.6801, -8.9383) (-81.0534, -9.9967) (-82.2692, -9.9704) (-82.2692, -10.3935) knots -1 -1 -1 -1 0 0 0 0
  spline S317 degree 3 poles (-82.2692, -10.3935) (-82.2692, -10.7109) (-81.9777, -11.2933) (-81.768, -11.2666) knots -1 -1 -1 -1 0 0 0 0
  spline S318 degree 3 poles (-81.768, -11.2666) (-81.3698, -11.2136) (-80.577, -11.1902) (-79.7806, -11.1902) knots -1 -1 -1 -1 0 0 0 0
  spline S319 degree 3 poles (-79.7806, -11.1902) (-78.9878, -11.1902) (-78.1951, -11.2136) (-77.772, -11.2666) knots -1 -1 -1 -1 0 0 0 0
  spline S320 degree 3 poles (-77.772, -11.2666) (-77.5587, -11.2933) (-77.2956, -10.7109) (-77.2956, -10.3935) knots -1 -1 -1 -1 0 0 0 0
  spline S321 degree 3 poles (-77.2956, -10.3935) (-77.2956, -9.9704) (-78.9629, -9.9967) (-78.5932, -8.9383) knots -1 -1 -1 -1 0 0 0 0
  line L81 (-78.5932, -8.9383) -> (-74.6506, 2.4388)
  line L82 (-74.6506, 2.4388) -> (-70.6626, -9.3268)
  spline S322 degree 3 poles (-70.6626, -9.3268) (-70.7276, -9.7127) (-71.1604, -9.8874) (-71.5166, -10.0352) knots -0.858522 -0.858522 -0.858522 -0.858522 -0.365068 -0.365068 -0.365068 -0.365068
  spline S323 degree 5 poles (-71.5166, -10.0352) (-71.5378, -10.0556) (-71.6088, -10.1255) (-71.7201, -10.2417) (-71.821, -10.3613) (-71.8986, -10.4733) (-71.9463, -10.562) (-71.967, -10.6087) (-71.9703, -10.6166) knots -0.740882 -0.740882 -0.740882 -0.740882 -0.740882 -0.740882 -0.7 -0.6 -0.5 -0.479543 -0.479543 -0.479543 -0.479543 -0.479543 -0.479543
  spline S324 degree 3 poles (-71.9703, -10.6166) (-71.9088, -10.861) (-71.7664, -11.1349) (-71.625, -11.231) knots -0.790921 -0.790921 -0.790921 -0.790921 -0.15171 -0.15171 -0.15171 -0.15171
  spline S325 degree 5 poles (-71.625, -11.231) (-71.6062, -11.2385) (-71.5869, -11.2458) (-71.567, -11.2529) (-71.5465, -11.2598) (-71.5256, -11.2666) knots -0.041035 -0.041035 -0.041035 -0.041035 -0.041035 -0.041035 0 0 0 0 0 0
  spline S326 degree 3 poles (-71.5256, -11.2666) (-70.4697, -11.2136) (-69.0939, -11.1902) (-67.7181, -11.1902) knots -1 -1 -1 -1 0 0 0 0
  spline S327 degree 3 poles (-67.7181, -11.1902) (-66.3422, -11.1902) (-64.9664, -11.2136) (-63.907, -11.2666) knots -1 -1 -1 -1 0 0 0 0
  spline S328 degree 5 poles (-63.907, -11.2666) (-63.8508, -11.2222) (-63.7825, -11.1656) (-63.7203, -11.1105) (-63.6642, -11.057) (-63.6143, -11.005) (-63.6031, -10.9931) knots -1 -1 -1 -1 -1 -1 -0.933333 -0.913312 -0.913312 -0.913312 -0.913312 -0.913312 -0.913312
  spline S329 degree 3 poles (-63.6031, -10.9931) (-63.4913, -10.8075) (-63.4057, -10.5655) (-63.4057, -10.3935) knots -0.541892 -0.541892 -0.541892 -0.541892 0 0 0 0
  spline S330 degree 5 poles (-63.4057, -10.3935) (-63.4069, -10.3913) (-63.4229, -10.3621) (-63.4609, -10.3077) (-63.5364, -10.2311) (-63.6683, -10.1358) (-63.8597, -10.0252) (-64.0239, -9.9353) (-64.1456, -9.8652) (-64.2235, -9.8172) (-64.2599, -9.7941) knots -0.672047 -0.672047 -0.672047 -0.672047 -0.672047 -0.672047 -0.666667 -0.6 -0.533333 -0.466667 -0.4 -0.340251 -0.340251 -0.340251 -0.340251 -0.340251 -0.340251
  spline S331 degree 3 poles (-64.2599, -9.7941) (-64.5406, -9.6256) (-64.8201, -9.3864) (-64.9744, -8.9843) knots -0.406295 -0.406295 -0.406295 -0.406295 -0.014693 -0.014693 -0.014693 -0.014693
  spline S332 degree 5 poles (-64.9744, -8.9843) (-64.9779, -8.9752) (-64.9814, -8.966) (-64.9848, -8.9569) (-64.9881, -8.9476) (-64.9913, -8.9383) knots -0.014784 -0.014784 -0.014784 -0.014784 -0.014784 -0.014784 0 0 0 0 0 0
  ellipse E16 centre (-49.574, -11.5198) end of major axis (-54.89, -11.5263) minor radius 0.3056 (-49.4642, -11.2142) -> (-53.0631, -11.2935) ccw
  ellipse E17 centre (-49.574, -11.5198) end of major axis (-54.89, -11.5263) minor radius 0.3056 (-49.4642, -11.2142) -> (-53.0631, -11.2935) ccw
  spline S333 degree 3 poles (-116.6669, -11.2934) (-117.725, -11.2403) (-119.2598, -11.2139) (-120.8217, -11.2139) knots 0 0 0 0 1 1 1 1
  spline S334 degree 3 poles (-120.8217, -11.2139) (-119.2598, -11.2139) (-117.725, -11.2403) (-116.6669, -11.2934) knots -1 -1 -1 -1 0 0 0 0
  spline S335 degree 3 poles (2.7113, 4.1848) (2.7113, 5.2959) (1.2548, 5.2165) (1.2548, 5.6398) knots 0 0 0 0 1 1 1 1
  spline S336 degree 3 poles (1.2548, 5.6398) (1.2548, 5.2165) (2.7113, 5.2959) (2.7113, 4.1848) knots -1 -1 -1 -1 0 0 0 0
  spline S337 degree 3 poles (-82.2692, -10.3935) (-82.2692, -9.9704) (-81.0534, -9.9967) (-80.6801, -8.9383) knots 0 0 0 0 1 1 1 1
  spline S338 degree 3 poles (-80.6801, -8.9383) (-81.0534, -9.9967) (-82.2692, -9.9704) (-82.2692, -10.3935) knots -1 -1 -1 -1 0 0 0 0
  spline S339 degree 3 poles (1.4134, -2.4299) (1.8367, -2.4299) (2.7113, -2.377) (2.7113, -3.0383) knots -1 -1 -1 -1 0 0 0 0
  spline S340 degree 3 poles (1.4134, -2.4299) (1.8367, -2.4299) (2.7113, -2.377) (2.7113, -3.0383) knots -1 -1 -1 -1 0 0 0 0
  spline S341 degree 3 poles (-2.6606, -5.949) (-2.6606, -3.8323) (-1.2321, -2.4299) (1.4134, -2.4299) knots -1 -1 -1 -1 0 0 0 0
  spline S342 degree 3 poles (-2.6606, -5.949) (-2.6606, -3.8323) (-1.2321, -2.4299) (1.4134, -2.4299) knots -1 -1 -1 -1 0 0 0 0
  spline S343 degree 5 poles (-64.2599, -9.7941) (-64.2235, -9.8172) (-64.1456, -9.8652) (-64.0239, -9.9353) (-63.8597, -10.0252) (-63.6683, -10.1358) (-63.5364, -10.2311) (-63.4609, -10.3077) (-63.4229, -10.3621) (-63.4069, -10.3913) (-63.4057, -10.3935) knots 0.340251 0.340251 0.340251 0.340251 0.340251 0.340251 0.4 0.466667 0.533333 0.6 0.666667 0.672047 0.672047 0.672047 0.672047 0.672047 0.672047
  spline S344 degree 5 poles (-63.4057, -10.3935) (-63.4069, -10.3913) (-63.4229, -10.3621) (-63.4609, -10.3077) (-63.5364, -10.2311) (-63.6683, -10.1358) (-63.8597, -10.0252) (-64.0239, -9.9353) (-64.1456, -9.8652) (-64.2235, -9.8172) (-64.2599, -9.7941) knots -0.672047 -0.672047 -0.672047 -0.672047 -0.672047 -0.672047 -0.666667 -0.6 -0.533333 -0.466667 -0.4 -0.340251 -0.340251 -0.340251 -0.340251 -0.340251 -0.340251
  spline S345 degree 3 poles (-46.7651, -8.9652) (-46.7651, -10.0765) (-45.3365, -9.9971) (-45.3365, -10.4202) knots 0 0 0 0 1 1 1 1
  spline S346 degree 3 poles (-45.3365, -10.4202) (-45.3365, -9.9971) (-46.7651, -10.0765) (-46.7651, -8.9652) knots -1 -1 -1 -1 0 0 0 0
  line L83 (-59.2547, -8.9652) -> (-59.2547, -0.3134)
  line L84 (-59.2547, -0.3134) -> (-59.2547, -8.9652)
  spline S347 degree 3 poles (-45.3365, -10.4202) (-45.3365, -10.7379) (-45.601, -11.2935) (-45.8379, -11.2935) knots 0 0 0 0 1 1 1 1
  spline S348 degree 3 poles (-45.8379, -11.2935) (-45.601, -11.2935) (-45.3365, -10.7379) (-45.3365, -10.4202) knots -1 -1 -1 -1 0 0 0 0
  spline S349 degree 3 poles (-71.5166, -10.0352) (-71.1604, -9.8874) (-70.7276, -9.7127) (-70.6626, -9.3268) knots 0.365068 0.365068 0.365068 0.365068 0.858522 0.858522 0.858522 0.858522
  spline S350 degree 3 poles (-70.6626, -9.3268) (-70.7276, -9.7127) (-71.1604, -9.8874) (-71.5166, -10.0352) knots -0.858522 -0.858522 -0.858522 -0.858522 -0.365068 -0.365068 -0.365068 -0.365068
  spline S351 degree 3 poles (-55.6798, 4.3435) (-57.9291, 4.3435) (-59.2547, 2.7559) (-59.2547, -0.3134) knots 0 0 0 0 1 1 1 1
  spline S352 degree 3 poles (-59.2547, -0.3134) (-59.2547, 2.7559) (-57.9291, 4.3435) (-55.6798, 4.3435) knots -1 -1 -1 -1 0 0 0 0
  spline S353 degree 3 poles (-75.2585, 6.5133) (-74.3591, 6.4603) (-73.5911, 6.434) (-72.8517, 6.434) knots 0 0 0 0 1 1 1 1
  spline S354 degree 3 poles (-72.8517, 6.434) (-73.5911, 6.434) (-74.3591, 6.4603) (-75.2585, 6.5133) knots -1 -1 -1 -1 0 0 0 0
  spline S355 degree 5 poles (-64.9913, -8.9383) (-64.9881, -8.9476) (-64.9848, -8.9569) (-64.9814, -8.966) (-64.9779, -8.9752) (-64.9744, -8.9843) knots 0 0 0 0 0 0 0.014784 0.014784 0.014784 0.014784 0.014784 0.014784
  spline S356 degree 5 poles (-64.9744, -8.9843) (-64.9779, -8.9752) (-64.9814, -8.966) (-64.9848, -8.9569) (-64.9881, -8.9476) (-64.9913, -8.9383) knots -0.014784 -0.014784 -0.014784 -0.014784 -0.014784 -0.014784 0 0 0 0 0 0
  ellipse E18 centre (-50.1303, -11.6956) end of major axis (-56.9584, -11.7428) minor radius 0.4792 (-45.8379, -11.2935) -> (-49.4642, -11.2142) ccw
  ellipse E19 centre (-50.1303, -11.6956) end of major axis (-56.9584, -11.7428) minor radius 0.4792 (-45.8379, -11.2935) -> (-49.4642, -11.2142) ccw
  line L85 (-70.4164, 6.5133) -> (-64.9913, -8.9383)
  spline S357 degree 5 poles (-64.9913, -8.9383) (-64.9881, -8.9476) (-64.9848, -8.9569) (-64.9814, -8.966) (-64.9779, -8.9752) (-64.9744, -8.9843) knots 0 0 0 0 0 0 0.014784 0.014784 0.014784 0.014784 0.014784 0.014784
  spline S358 degree 3 poles (-64.9744, -8.9843) (-64.8201, -9.3864) (-64.5406, -9.6256) (-64.2599, -9.7941) knots 0.014693 0.014693 0.014693 0.014693 0.406295 0.406295 0.406295 0.406295
  spline S359 degree 5 poles (-64.2599, -9.7941) (-64.2235, -9.8172) (-64.1456, -9.8652) (-64.0239, -9.9353) (-63.8597, -10.0252) (-63.6683, -10.1358) (-63.5364, -10.2311) (-63.4609, -10.3077) (-63.4229, -10.3621) (-63.4069, -10.3913) (-63.4057, -10.3935) knots 0.340251 0.340251 0.340251 0.340251 0.340251 0.340251 0.4 0.466667 0.533333 0.6 0.666667 0.672047 0.672047 0.672047 0.672047 0.672047 0.672047
  spline S360 degree 3 poles (-63.4057, -10.3935) (-63.4057, -10.5655) (-63.4913, -10.8075) (-63.6031, -10.9931) knots 0 0 0 0 0.541892 0.541892 0.541892 0.541892
  spline S361 degree 5 poles (-63.6031, -10.9931) (-63.6143, -11.005) (-63.6642, -11.057) (-63.7203, -11.1105) (-63.7825, -11.1656) (-63.8508, -11.2222) (-63.907, -11.2666) knots 0.913312 0.913312 0.913312 0.913312 0.913312 0.913312 0.933333 1 1 1 1 1 1
  spline S362 degree 3 poles (-63.907, -11.2666) (-64.9664, -11.2136) (-66.3422, -11.1902) (-67.7181, -11.1902) knots 0 0 0 0 1 1 1 1
  spline S363 degree 3 poles (-67.7181, -11.1902) (-69.0939, -11.1902) (-70.4697, -11.2136) (-71.5256, -11.2666) knots 0 0 0 0 1 1 1 1
  spline S364 degree 5 poles (-71.5256, -11.2666) (-71.5465, -11.2598) (-71.567, -11.2529) (-71.5869, -11.2458) (-71.6062, -11.2385) (-71.625, -11.231) knots 0 0 0 0 0 0 0.041035 0.041035 0.041035 0.041035 0.041035 0.041035
  spline S365 degree 3 poles (-71.625, -11.231) (-71.7664, -11.1349) (-71.9088, -10.861) (-71.9703, -10.6166) knots 0.15171 0.15171 0.15171 0.15171 0.790921 0.790921 0.790921 0.790921
  spline S366 degree 5 poles (-71.9703, -10.6166) (-71.967, -10.6087) (-71.9463, -10.562) (-71.8986, -10.4733) (-71.821, -10.3613) (-71.7201, -10.2417) (-71.6088, -10.1255) (-71.5378, -10.0556) (-71.5166, -10.0352) knots 0.479543 0.479543 0.479543 0.479543 0.479543 0.479543 0.5 0.6 0.7 0.740882 0.740882 0.740882 0.740882 0.740882 0.740882
  spline S367 degree 3 poles (-71.5166, -10.0352) (-71.1604, -9.8874) (-70.7276, -9.7127) (-70.6626, -9.3268) knots 0.365068 0.365068 0.365068 0.365068 0.858522 0.858522 0.858522 0.858522
  line L86 (-70.6626, -9.3268) -> (-74.6506, 2.4388)
  line L87 (-74.6506, 2.4388) -> (-78.5932, -8.9383)
  spline S368 degree 3 poles (-78.5932, -8.9383) (-78.9629, -9.9967) (-77.2956, -9.9704) (-77.2956, -10.3935) knots 0 0 0 0 1 1 1 1
  spline S369 degree 3 poles (-77.2956, -10.3935) (-77.2956, -10.7109) (-77.5587, -11.2933) (-77.772, -11.2666) knots 0 0 0 0 1 1 1 1
  spline S370 degree 3 poles (-77.772, -11.2666) (-78.1951, -11.2136) (-78.9878, -11.1902) (-79.7806, -11.1902) knots 0 0 0 0 1 1 1 1
  spline S371 degree 3 poles (-79.7806, -11.1902) (-80.577, -11.1902) (-81.3698, -11.2136) (-81.768, -11.2666) knots 0 0 0 0 1 1 1 1
  spline S372 degree 3 poles (-81.768, -11.2666) (-81.9777, -11.2933) (-82.2692, -10.7109) (-82.2692, -10.3935) knots 0 0 0 0 1 1 1 1
  spline S373 degree 3 poles (-82.2692, -10.3935) (-82.2692, -9.9704) (-81.0534, -9.9967) (-80.6801, -8.9383) knots 0 0 0 0 1 1 1 1
  line L88 (-80.6801, -8.9383) -> (-75.2585, 6.5133)
  spline S374 degree 3 poles (-75.2585, 6.5133) (-74.3591, 6.4603) (-73.5911, 6.434) (-72.8517, 6.434) knots 0 0 0 0 1 1 1 1
  spline S375 degree 3 poles (-72.8517, 6.434) (-72.0838, 6.434) (-71.3407, 6.4603) (-70.4164, 6.5133) knots 0 0 0 0 1 1 1 1
  spline S376 degree 3 poles (310.3894, -11.2934) (308.5106, -11.1346) (306.4998, -11.2934) (305.5999, -11.2934) knots 0 0 0 0 1 1 1 1
  spline S377 degree 3 poles (305.5999, -11.2934) (306.4998, -11.2934) (308.5106, -11.1346) (310.3894, -11.2934) knots -1 -1 -1 -1 0 0 0 0
  spline S378 degree 3 poles (-125.4494, -10.4202) (-125.4494, -10.0233) (-123.651, -9.9175) (-124.2866, -8.9652) knots 0 0 0 0 1 1 1 1
  line L89 (-124.2866, -8.9652) -> (-127.1702, -4.5202)
  line L90 (-127.1702, -4.5202) -> (-130.0537, -8.9121)
  spline S379 degree 3 poles (-130.0537, -8.9121) (-130.6622, -9.8648) (-129.1545, -9.9969) (-129.1545, -10.4202) knots 0 0 0 0 1 1 1 1
  spline S380 degree 3 poles (-129.1545, -10.4202) (-129.1545, -10.7376) (-129.5266, -11.3224) (-129.7359, -11.2934) knots 0 0 0 0 1 1 1 1
  spline S381 degree 3 poles (-129.7359, -11.2934) (-130.1351, -11.2403) (-130.8754, -11.2139) (-131.6156, -11.2139) knots 0 0 0 0 1 1 1 1
  spline S382 degree 3 poles (-131.6156, -11.2139) (-132.3559, -11.2139) (-133.0961, -11.2403) (-133.4953, -11.2934) knots 0 0 0 0 1 1 1 1
  spline S383 degree 3 poles (-133.4953, -11.2934) (-133.7046, -11.3224) (-133.9953, -10.7376) (-133.9953, -10.4202) knots 0 0 0 0 1 1 1 1
  spline S384 degree 3 poles (-133.9953, -10.4202) (-133.9953, -9.9969) (-133.0729, -9.8648) (-132.4373, -8.9121) knots 0 0 0 0 1 1 1 1
  line L91 (-132.4373, -8.9121) -> (-128.3096, -2.7738)
  line L92 (-128.3096, -2.7738) -> (-132.8326, 4.1584)
  spline S385 degree 3 poles (-132.8326, 4.1584) (-133.4411, 5.1106) (-134.5263, 5.2164) (-134.5263, 5.64) knots 0 0 0 0 1 1 1 1
  spline S386 degree 3 poles (-134.5263, 5.64) (-134.5263, 5.9575) (-134.2356, 6.5132) (-134.0225, 6.5132) knots 0 0 0 0 1 1 1 1
  spline S387 degree 3 poles (-134.0225, 6.5132) (-132.9915, 6.4601) (-131.4296, 6.4338) (-129.8948, 6.4338) knots 0 0 0 0 1 1 1 1
  spline S388 degree 3 poles (-129.8948, 6.4338) (-128.3368, 6.4338) (-126.802, 6.4601) (-125.7439, 6.5132) knots 0 0 0 0 1 1 1 1
  spline S389 degree 3 poles (-125.7439, 6.5132) (-125.5308, 6.5132) (-125.2401, 5.9575) (-125.2401, 5.64) knots 0 0 0 0 1 1 1 1
  spline S390 degree 3 poles (-125.2401, 5.64) (-125.2401, 5.2164) (-127.0384, 5.1106) (-126.4299, 4.1584) knots 0 0 0 0 1 1 1 1
  line L93 (-126.4299, 4.1584) -> (-122.9922, -1.0805)
  line L94 (-122.9922, -1.0805) -> (-119.6048, 4.132)
  spline S391 degree 3 poles (-119.6048, 4.132) (-118.9691, 5.0843) (-120.4768, 5.2164) (-120.4768, 5.6133) knots 0 0 0 0 1 1 1 1
  spline S392 degree 3 poles (-120.4768, 5.6133) (-120.4768, 5.9311) (-120.1048, 6.5396) (-119.8955, 6.5132) knots 0 0 0 0 1 1 1 1
  spline S393 degree 3 poles (-119.8955, 6.5132) (-119.4963, 6.4601) (-118.756, 6.4338) (-118.0157, 6.4338) knots 0 0 0 0 1 1 1 1
  spline S394 degree 3 poles (-118.0157, 6.4338) (-117.2755, 6.4338) (-116.5352, 6.4601) (-116.136, 6.5132) knots 0 0 0 0 1 1 1 1
  spline S395 degree 3 poles (-116.136, 6.5132) (-115.9267, 6.5396) (-115.636, 5.9311) (-115.636, 5.6133) knots 0 0 0 0 1 1 1 1
  spline S396 degree 3 poles (-115.636, 5.6133) (-115.636, 5.2164) (-116.5623, 5.0843) (-117.1979, 4.132) knots 0 0 0 0 1 1 1 1
  line L95 (-117.1979, 4.132) -> (-121.8798, -2.8001)
  line L96 (-121.8798, -2.8001) -> (-117.8839, -8.9652)
  spline S397 degree 3 poles (-117.8839, -8.9652) (-117.2483, -9.9175) (-116.1631, -9.9969) (-116.1631, -10.4202) knots 0 0 0 0 1 1 1 1
  spline S398 degree 3 poles (-116.1631, -10.4202) (-116.1631, -10.7376) (-116.4538, -11.3224) (-116.6669, -11.2934) knots 0 0 0 0 1 1 1 1
  spline S399 degree 3 poles (-116.6669, -11.2934) (-117.725, -11.2403) (-119.2598, -11.2139) (-120.8217, -11.2139) knots 0 0 0 0 1 1 1 1
  spline S400 degree 3 poles (-120.8217, -11.2139) (-122.3565, -11.2139) (-123.9184, -11.2403) (-124.9494, -11.2934) knots 0 0 0 0 1 1 1 1
  spline S401 degree 3 poles (-124.9494, -11.2934) (-125.1587, -11.3224) (-125.4494, -10.7376) (-125.4494, -10.4202) knots 0 0 0 0 1 1 1 1
  line L97 (175.9039, -3.885) -> (182.2539, -3.885)
  line L98 (182.2539, -3.885) -> (175.9039, -3.885)
  spline S402 degree 3 poles (-125.4494, -10.4202) (-125.4494, -10.0233) (-123.651, -9.9175) (-124.2866, -8.9652) knots 0 0 0 0 1 1 1 1
  spline S403 degree 3 poles (-124.2866, -8.9652) (-123.651, -9.9175) (-125.4494, -10.0233) (-125.4494, -10.4202) knots -1 -1 -1 -1 0 0 0 0
  spline S404 degree 3 poles (-4.0362, -1.0807) (-6.0748, -0.3396) (-6.9463, 1.9358) (-8.269, 4.1319) knots 0 0 0 0 1 1 1 1
  spline S405 degree 3 poles (-8.269, 4.1319) (-6.9463, 1.9358) (-6.0748, -0.3396) (-4.0362, -1.0807) knots -1 -1 -1 -1 0 0 0 0
  spline S406 degree 3 poles (-62.5342, -10.4202) (-62.5342, -9.9971) (-61.1571, -10.0765) (-61.1571, -8.9652) knots 0 0 0 0 1 1 1 1
  spline S407 degree 3 poles (-61.1571, -8.9652) (-61.1571, -10.0765) (-62.5342, -9.9971) (-62.5342, -10.4202) knots -1 -1 -1 -1 0 0 0 0
  spline S408 degree 3 poles (5.3848, 6.4338) (6.6827, 6.4338) (7.9525, 6.4602) (9.0107, 6.5131) knots 0 0 0 0 1 1 1 1
  spline S409 degree 3 poles (9.0107, 6.5131) (7.9525, 6.4602) (6.6827, 6.4338) (5.3848, 6.4338) knots -1 -1 -1 -1 0 0 0 0
  spline S410 degree 3 poles (-81.768, -11.2666) (-81.9777, -11.2933) (-82.2692, -10.7109) (-82.2692, -10.3935) knots 0 0 0 0 1 1 1 1
  spline S411 degree 3 poles (-82.2692, -10.3935) (-82.2692, -10.7109) (-81.9777, -11.2933) (-81.768, -11.2666) knots -1 -1 -1 -1 0 0 0 0
  line L99 (2.7113, -3.0383) -> (2.7113, -9.4149)
  line L100 (2.7113, -9.4149) -> (2.7113, -3.0383)
  line L101 (1.3605, -9.4149) -> (2.7113, -9.4149)
  line L102 (2.7113, -9.4149) -> (2.7113, -3.0383)
  spline S412 degree 3 poles (1.4134, -2.4299) (1.8367, -2.4299) (2.7113, -2.377) (2.7113, -3.0383) knots -1 -1 -1 -1 0 0 0 0
  spline S413 degree 3 poles (-2.6606, -5.949) (-2.6606, -3.8323) (-1.2321, -2.4299) (1.4134, -2.4299) knots -1 -1 -1 -1 0 0 0 0
  spline S414 degree 3 poles (1.3605, -9.4149) (-1.285, -9.4149) (-2.6606, -8.0125) (-2.6606, -5.949) knots -1 -1 -1 -1 0 0 0 0
  spline S415 degree 3 poles (9.5118, 5.6398) (9.5118, 5.2165) (8.0583, 5.2959) (8.0583, 4.1848) knots 0 0 0 0 1 1 1 1
  line L103 (8.0583, 4.1848) -> (8.0583, -8.9652)
  spline S416 degree 3 poles (8.0583, -8.9652) (8.0583, -10.0763) (9.5118, -9.9969) (9.5118, -10.4202) knots 0 0 0 0 1 1 1 1
  spline S417 degree 3 poles (9.5118, -10.4202) (9.5118, -10.738) (9.2223, -11.3225) (9.0107, -11.2935) knots 0 0 0 0 1 1 1 1
  spline S418 degree 3 poles (9.0107, -11.2935) (7.9525, -11.2406) (6.6827, -11.2142) (5.5155, -11.2142) knots 0 0 0 0 1 1 1 1
  spline S419 degree 3 poles (5.5155, -11.2142) (3.6357, -11.2142) (3.2124, -11.2935) (0.4331, -11.2935) knots 0 0 0 0 1 1 1 1
  spline S420 degree 3 poles (0.4331, -11.2935) (-5.0695, -11.2935) (-8.5087, -9.2826) (-8.5087, -5.8961) knots 0 0 0 0 1 1 1 1
  spline S421 degree 3 poles (-8.5087, -5.8961) (-8.5087, -3.5677) (-6.8685, -1.9008) (-4.0362, -1.0807) knots 0 0 0 0 1 1 1 1
  spline S422 degree 3 poles (-4.0362, -1.0807) (-6.0748, -0.3396) (-6.9463, 1.9358) (-8.269, 4.1319) knots 0 0 0 0 1 1 1 1
  spline S423 degree 3 poles (-8.269, 4.1319) (-8.851, 5.1107) (-10.096, 5.2165) (-10.096, 5.6134) knots 0 0 0 0 1 1 1 1
  spline S424 degree 3 poles (-10.096, 5.6134) (-10.096, 5.9308) (-9.8034, 6.5131) (-9.5918, 6.5131) knots 0 0 0 0 1 1 1 1
  spline S425 degree 3 poles (-9.5918, 6.5131) (-6.3923, 6.328) (-4.9108, 6.4867) (-4.0362, 6.4867) knots 0 0 0 0 1 1 1 1
  spline S426 degree 3 poles (-4.0362, 6.4867) (-2.3431, 6.4867) (-3.3764, 5.8779) (-2.1844, 4.1319) knots 0 0 0 0 1 1 1 1
  line L104 (-2.1844, 4.1319) -> (0.9622, -0.5248)
  line L105 (0.9622, -0.5248) -> (2.7113, -0.5248)
  line L106 (2.7113, -0.5248) -> (2.7113, 4.1848)
  spline S427 degree 3 poles (2.7113, 4.1848) (2.7113, 5.2959) (1.2548, 5.2165) (1.2548, 5.6398) knots 0 0 0 0 1 1 1 1
  spline S428 degree 3 poles (1.2548, 5.6398) (1.2548, 5.9573) (1.5442, 6.5131) (1.7558, 6.5131) knots 0 0 0 0 1 1 1 1
  spline S429 degree 3 poles (1.7558, 6.5131) (2.7891, 6.4602) (4.087, 6.4338) (5.3848, 6.4338) knots 0 0 0 0 1 1 1 1
  spline S430 degree 3 poles (5.3848, 6.4338) (6.6827, 6.4338) (7.9525, 6.4602) (9.0107, 6.5131) knots 0 0 0 0 1 1 1 1
  spline S431 degree 3 poles (9.0107, 6.5131) (9.2223, 6.5131) (9.5118, 5.9573) (9.5118, 5.6398) knots 0 0 0 0 1 1 1 1
  spline S432 degree 3 poles (1.2548, 5.6398) (1.2548, 5.9573) (1.5442, 6.5131) (1.7558, 6.5131) knots 0 0 0 0 1 1 1 1
  spline S433 degree 3 poles (1.7558, 6.5131) (1.5442, 6.5131) (1.2548, 5.9573) (1.2548, 5.6398) knots -1 -1 -1 -1 0 0 0 0
  spline S434 degree 3 poles (-64.9744, -8.9843) (-64.8201, -9.3864) (-64.5406, -9.6256) (-64.2599, -9.7941) knots 0.014693 0.014693 0.014693 0.014693 0.406295 0.406295 0.406295 0.406295
  spline S435 degree 3 poles (-64.2599, -9.7941) (-64.5406, -9.6256) (-64.8201, -9.3864) (-64.9744, -8.9843) knots -0.406295 -0.406295 -0.406295 -0.406295 -0.014693 -0.014693 -0.014693 -0.014693
  spline S436 degree 3 poles (-77.772, -11.2666) (-78.1951, -11.2136) (-78.9878, -11.1902) (-79.7806, -11.1902) knots 0 0 0 0 1 1 1 1
  spline S437 degree 3 poles (-79.7806, -11.1902) (-78.9878, -11.1902) (-78.1951, -11.2136) (-77.772, -11.2666) knots -1 -1 -1 -1 0 0 0 0
  spline S438 degree 3 poles (-63.907, -11.2666) (-64.9664, -11.2136) (-66.3422, -11.1902) (-67.7181, -11.1902) knots 0 0 0 0 1 1 1 1
  spline S439 degree 3 poles (-67.7181, -11.1902) (-66.3422, -11.1902) (-64.9664, -11.2136) (-63.907, -11.2666) knots -1 -1 -1 -1 0 0 0 0
  spline S440 degree 3 poles (-77.2956, -10.3935) (-77.2956, -10.7109) (-77.5587, -11.2933) (-77.772, -11.2666) knots 0 0 0 0 1 1 1 1
  spline S441 degree 3 poles (-77.772, -11.2666) (-77.5587, -11.2933) (-77.2956, -10.7109) (-77.2956, -10.3935) knots -1 -1 -1 -1 0 0 0 0
  spline S442 degree 3 poles (-67.7181, -11.1902) (-69.0939, -11.1902) (-70.4697, -11.2136) (-71.5256, -11.2666) knots 0 0 0 0 1 1 1 1
  spline S443 degree 3 poles (-71.5256, -11.2666) (-70.4697, -11.2136) (-69.0939, -11.1902) (-67.7181, -11.1902) knots -1 -1 -1 -1 0 0 0 0
  spline S444 degree 3 poles (-78.5932, -8.9383) (-78.9629, -9.9967) (-77.2956, -9.9704) (-77.2956, -10.3935) knots 0 0 0 0 1 1 1 1
  spline S445 degree 3 poles (-77.2956, -10.3935) (-77.2956, -9.9704) (-78.9629, -9.9967) (-78.5932, -8.9383) knots -1 -1 -1 -1 0 0 0 0
  spline S446 degree 3 poles (189.0272, 5.64) (189.0272, 5.2166) (187.5984, 5.296) (187.5984, 4.1583) knots 0 0 0 0 1 1 1 1
  spline S447 degree 3 poles (187.5984, 4.1583) (187.5984, 5.296) (189.0272, 5.2166) (189.0272, 5.64) knots -1 -1 -1 -1 0 0 0 0
  line L107 (-117.8839, -8.9652) -> (-121.8798, -2.8001)
  line L108 (-121.8798, -2.8001) -> (-117.8839, -8.9652)
  spline S448 degree 3 poles (163.9182, -11.214) (162.6218, -11.214) (161.3253, -11.2405) (160.2934, -11.2934) knots 0 0 0 0 1 1 1 1
  spline S449 degree 3 poles (160.2934, -11.2934) (161.3253, -11.2405) (162.6218, -11.214) (163.9182, -11.214) knots -1 -1 -1 -1 0 0 0 0
  spline S450 degree 3 poles (1.7558, 6.5131) (2.7891, 6.4602) (4.087, 6.4338) (5.3848, 6.4338) knots 0 0 0 0 1 1 1 1
  spline S451 degree 3 poles (5.3848, 6.4338) (4.087, 6.4338) (2.7891, 6.4602) (1.7558, 6.5131) knots -1 -1 -1 -1 0 0 0 0
  spline S452 degree 3 poles (-11.8921, 6.5129) (-11.5493, 6.5129) (-11.3378, 6.1954) (-11.2033, 5.6928) knots 0 0 0 0 1 1 1 1
  spline S453 degree 3 poles (-11.2033, 5.6928) (-11.3378, 6.1954) (-11.5493, 6.5129) (-11.8921, 6.5129) knots -1 -1 -1 -1 0 0 0 0
  line L109 (311.8446, 1.6183) -> (305.6267, 1.5654)
  line L110 (305.6267, 1.5654) -> (311.8446, 1.6183)
  spline S454 degree 3 poles (176.8564, -11.2934) (175.798, -11.2405) (174.5016, -11.214) (173.2316, -11.214) knots 0 0 0 0 1 1 1 1
  spline S455 degree 3 poles (173.2316, -11.214) (174.5016, -11.214) (175.798, -11.2405) (176.8564, -11.2934) knots -1 -1 -1 -1 0 0 0 0
  line L111 (-121.8798, -2.8001) -> (-117.1979, 4.132)